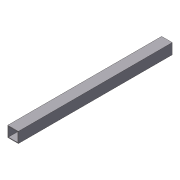
# Autodesk Inventor part: Frame_LowerConveyorBallSupport
Saved by Autodesk Inventor 2012 (Build 160160000, 160)
## iProperties
Created: 2012-01-19
Part Number: Frame_LowerConveyorBallSupport
Material: Aluminum-6061
Document SubType Name: Modeling
Designer: JesseK
Mass: 150.921 g
Surface Area: 704.636 cm^2
Volume: 55.6904 cm^3
Density: 2.71 g/cm^3
Author: JesseK
Autodesk Inventor part; units mm, degrees
ref_plane "YZ Plane" through (0, 0, 0) normal (1, 0, 0) x (0, 1, 0)
ref_plane "XZ Plane" through (0, 0, 0) normal (0, 1, 0) x (-1, 0, 0)
ref_plane "XY Plane" through (0, 0, 0) normal (0, 0, 1) x (1, 0, 0)
sketch "Sketch1" plane through (0, 0, 0) normal (0, 0, 1) x (1, 0, 0)
  line L0 (0.1582, 137.0969) -> (-25.2418, 137.0969)
  line L1 (-25.2418, 137.0969) -> (-25.2418, 162.4969)
  line L2 (-25.2418, 162.4969) -> (0.1582, 162.4969)
  line L3 (0.1582, 162.4969) -> (0.1582, 137.0969)
  point P0 (0, 0)
  dimension "d0" = 25.4
  dimension "d1" = 25.4
  constraints: 8 end point, 2 parallel, 1 horizontal, 1 perpendicular
  measures "d0" distance of L0.start L0.end
  measures "d1" distance of L0.end L1.end
extrude "Extrusion1" add sketch "Sketch1" along normal blind 368.3
shell "Shell1" thickness 1.5875 removed faces 2 at (-8.3084, 145.5636, 0) at (-8.3084, 145.5636, 368.3)
body "Solid1"
